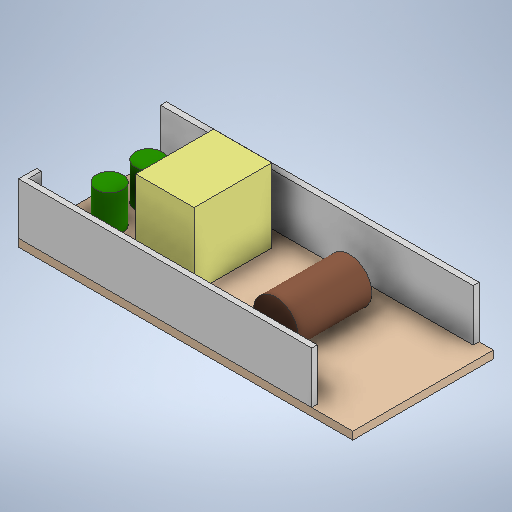
# Autodesk Inventor part: 12vconverter
Saved by Autodesk Inventor 2025 (Build 290162000, 162)
## iProperties
Created: 2025-05-12
Part Number: 12vconverter
Material: Generic
Document SubType Name: Modeling
Designer: ethan
Density: 1 g/cm^3
Appearance: Default
Author: ethan
Autodesk Inventor part; units mm, degrees
ref_plane "YZ Plane" through (0, 0, 0) normal (1, 0, 0) x (0, 1, 0)
ref_plane "XZ Plane" through (0, 0, 0) normal (0, 1, 0) x (-1, 0, 0)
ref_plane "XY Plane" through (0, 0, 0) normal (0, 0, 1) x (1, 0, 0)
sketch "Sketch1" plane through (0, 0, 0) normal (0, 1, 0) x (-1, 0, 0)
  line L0 (0, 0) -> (-109.22, 0)
  line L1 (-109.22, 0) -> (-109.22, -45.974)
  line L2 (-109.22, -45.974) -> (0, -45.974)
  line L3 (0, -45.974) -> (0, 0)
  dimension "d0" = 109.22
  dimension "d1" = 45.974
  constraints: 8 end point, 2 parallel, 1 horizontal, 1 perpendicular
  measures "d0" distance of L2.end L1.end
  measures "d1" distance of L1.end L0.end
extrude "Extrusion1" add sketch "Sketch1" along normal blind 2.54
sketch "Sketch2" plane through (0, 2.54, 0) normal (0, 1, 0) x (1, 0, 0)
  line L0 (109.22, 0) -> (109.22, 45.974) projected
  line L1 (109.22, 45.974) -> (0, 45.974) projected
  line L2 (0, 45.974) -> (0, 0) projected
  line L3 (0, 0) -> (109.22, 0) projected
  line L4 (2.3641, 45.974) -> (104.5271, 45.974)
  line L5 (104.5271, 45.974) -> (104.5271, 44.0473)
  line L6 (104.5271, 44.0473) -> (2.3641, 44.0473)
  line L7 (2.3641, 44.0473) -> (2.3641, 45.974)
  line L8 (0, 5.8755) -> (1.5541, 5.8755)
  line L9 (1.5541, 5.8755) -> (1.5541, 0)
  line L10 (1.5541, 0) -> (0, 0)
  line L11 (0, 0) -> (0, 5.8755)
  line L12 (0, 0) -> (95.8194, 0)
  line L13 (95.8194, 0) -> (95.8194, 1.8254)
  line L14 (95.8194, 1.8254) -> (0, 1.8254)
  line L15 (0, 1.8254) -> (0, 0)
  point P0 (1.5541, 1.8254)
  constraints: 24 end point, 6 parallel, 3 horizontal, 3 perpendicular, 3 point on line
extrude "Extrusion2" add sketch "Sketch2" along normal blind 16.8275 separate body contours L3 L9 L14 L13 | L5 L6 L7 L1 | L3 L2 L14 L9 | L14 L2 L8 L9
sketch "Sketch3" plane through (0, 2.54, 0) normal (0, 1, 0) x (1, 0, 0)
  circle A0 centre (11.0685, 31.4708) radius 4.3739
  circle A1 centre (11.0685, 18.6677) radius 4.2928
  point P0 (0, 0)
  constraints: 2 centre point
extrude "Extrusion3" add sketch "Sketch3" along normal blind 12.065 bodies 1
sketch "Sketch4" plane through (0, 2.54, 0) normal (0, 1, 0) x (1, 0, 0)
  circle A0 centre (11.0685, 18.6677) radius 4.2928 projected
  circle A1 centre (11.0685, 31.4708) radius 4.3739 projected
  line L0 (0, 0) -> (109.22, 0) projected
  line L1 (109.22, 0) -> (109.22, 45.974) projected
  line L2 (109.22, 45.974) -> (0, 45.974) projected
  line L3 (0, 45.974) -> (0, 0) projected
  line L4 (44.1347, 38.6247) -> (25.0847, 38.6247)
  line L5 (25.0847, 38.6247) -> (25.0847, 13.2247)
  line L6 (25.0847, 13.2247) -> (44.1347, 13.2247)
  line L7 (44.1347, 13.2247) -> (44.1347, 38.6247)
  line L8 (44.1347, 38.6247) -> (25.0847, 13.2247) construction
  line L9 (25.0847, 38.6247) -> (44.1347, 13.2247) construction
  point P0 (34.6097, 25.9247)
  dimension "d8" = 19.05
  dimension "d9" = 25.4
  constraints: 12 end point, 2 midpoint, 2 parallel, 1 horizontal, 1 perpendicular
  measures "d8" distance of L6.end L5.end
  measures "d9" distance of L5.end L4.end
extrude "Extrusion4" add sketch "Sketch4" along normal blind 24.13 contours L7 L6 L5 L4 bodies 1
ref_plane "Work Plane1" through (2.3641, 2.54, -22.9364) normal (0, 0, 1) x (1, 0, 0)
sketch "Sketch5" plane through (2.3641, 2.54, -22.9364) normal (0, 0, 1) x (1, 0, 0)
  line L0 (22.7205, 0) -> (41.7705, 0) projected
  line L1 (41.7705, 0) -> (22.7205, 0) projected
  line L2 (4.4115, 0) -> (12.9972, 0) projected
  line L3 (4.3304, 0) -> (13.0783, 0) projected
  line L4 (-2.3641, 0) -> (106.8559, 0) projected
  line L5 (106.8559, 0) -> (-2.3641, 0) projected
  circle A0 centre (70.7868, 7.2548) radius 7.2548
  line L6 (102.1629, 0) -> (0, 0) projected
  point P0 (-2.3641, -2.54)
  point P1 (93.4553, 0)
  point P2 (93.4553, 0)
  constraints: 1 centre point, 2 other
extrude "Extrusion5" add sketch "Sketch5" along normal mid plane 24.13 bodies 1
body "Solid1"
body "Solid2"
